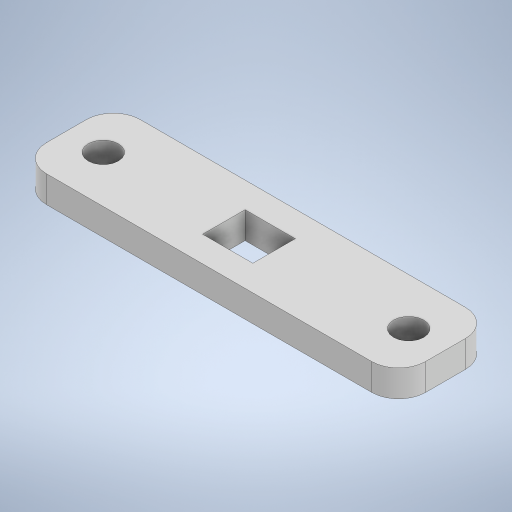
# Autodesk Inventor part: Spojovaci_clen
Saved by Autodesk Inventor 2024.2 (Build 282272000, 272)
## iProperties
Created: 2025-06-03
Part Number: Spojovaci_clen
Material: Všeobecné
Document SubType Name: Modeling
Designer: Elite
Density: 1 g/cm^3
Appearance: Výchozí
Author: Elite
Autodesk Inventor part; units mm, degrees
ref_plane "YZ Plane" through (0, 0, 0) normal (1, 0, 0) x (0, 1, 0)
ref_plane "XZ Plane" through (0, 0, 0) normal (0, 1, 0) x (-1, 0, 0)
ref_plane "XY Plane" through (0, 0, 0) normal (0, 0, 1) x (1, 0, 0)
sketch "Náčrt1" plane through (0, 0, 0) normal (0, 0, 1) x (1, 0, 0)
  line L0 (30.6144, 11.0767) -> (33.1544, 11.0767)
  line L1 (33.1544, 11.0767) -> (25.6544, 11.0767)
  line L2 (25.6544, 11.0767) -> (25.6544, 4.7267)
  line L3 (25.6544, 4.7267) -> (33.1544, 4.7267)
  line L4 (33.1544, 4.7267) -> (33.1544, 11.0767)
  line L5 (58.7544, 14.9017) -> (2.1544, 14.9017)
  circle A0 centre (7.6544, 7.9017) radius 2.25
  line L6 (2.1544, 14.9017) -> (2.1544, 0.9017)
  circle A1 centre (53.2544, 7.9017) radius 2.25
  line L7 (2.1544, 0.9017) -> (58.7544, 0.9017)
  line L8 (58.7544, 0.9017) -> (58.7544, 14.9017)
  point P0 (33.1544, 4.7267)
  point P1 (7.6544, 7.9017)
  point P2 (53.2544, 7.9017)
  dimension "d2" = 7.5
  dimension "d3" = 6.35
  constraints: 18 end point, 2 centre point, 2 parallel, 1 horizontal, 1 perpendicular
  measures "d2" distance of L0.end L1.end
  measures "d3" distance of L3.end L0.end
extrude "Vysunutí1" add sketch "Náčrt1" along normal blind 4
fillet "Zaoblení1" radius 4 4 edges at (58.7544, 0.9017, 2) (58.7544, 14.9017, 2) (2.1544, 14.9017, 2) (2.1544, 0.9017, 2)
